nixal_reprap_XmotorCompatible (Autodesk Fusion 360 design; units mm, degrees)
Autodesk Fusion 360 part; units mm, degrees
sketch "Sketch1" plane through (0, 0, 0) normal (0, 1, 0) x (1, 0, 0)
  circle A0 centre (0, 0) radius 4
  circle A1 centre (21, -2) radius 4
  circle A2 centre (21, -2) radius 13
  circle A3 centre (21, -2) radius 8 construction
  circle A4 centre (13, -1.9989) radius 1.8
  circle A5 centre (29, -2.0036) radius 1.8
  line L0 (21, -2) -> (21, 11) construction
  line L1 (21, -2) -> (34, -2) construction
  line L2 (41, 31) -> (-24, 31)
  line L3 (41, 31) -> (41, -15)
  circle A6 centre (0, 0) radius 6
  circle A7 centre (0, 0) radius 10.5
  line L4 (40.8805, 9) -> (-49.1195, 9)
  line L5 (-49.1195, 9) -> (-49.1195, 26)
  line L6 (-49.1195, 26) -> (40.8805, 26)
  line L7 (40.8805, 26) -> (40.8805, 9)
  line L8 (-10.5, 0.0002) -> (-10.4998, 9)
  line L9 (34, -2) -> (34, 9)
  line L10 (0, 0) -> (7.1243, -7.7132)
  line L11 (0, 0) -> (6, -9)
  circle A8 centre (21, -2) radius 5.5
  line L12 (10.5, 0.0203) -> (10.4826, 9)
  line L13 (7.1243, -7.7132) -> (14.0549, -12.9894)
  circle A9 centre (21, 6) radius 1.8
  circle A10 centre (20.9776, -10) radius 1.8
  dimension "d1" = 8
  dimension "d2" = 8
  dimension "d23" = 26
  dimension "d104" = 16
  dimension "d107" = 3.6
  dimension "d108" = 3.6
  dimension "d134" = 33
  dimension "d136" = 31
  dimension "d137" = 20
  dimension "d138" = 41
  dimension "d139" = 12
  dimension "d140" = 21
  dimension "d141" = 17
  dimension "d142" = 90
  dimension "d143" = 5
  dimension "d146" = 11
  dimension "d203" = 3.6
  dimension "d204" = 3.6
  constraint coincident A0.centre A6.centre
  constraint concentric A1 A2
  constraint coincident A3 A0.centre
  constraint coincident A3
  constraint coincident A2 A0.centre
  constraint vertical L0
  constraint horizontal L1
  constraint horizontal L2
  constraint vertical L3
  constraint concentric A0 A6
  constraint concentric A6 A7
  constraint horizontal L4
  constraint vertical L5
  constraint horizontal L6
  constraint vertical L7
  constraint coincident A7 A0.centre
  constraint coincident L4
  constraint tangent A7 L8
  constraint tangent A2 L9
  constraint concentric A3 A8
  constraint tangent A7 L12
  constraint coincident L0 A0.centre
  measures "d1" diameter of A0
  measures "d2" diameter of A1
  measures "d23" diameter of A2
  measures "d104" diameter of A3
  measures "d107" diameter of A4
  measures "d108" diameter of A5
  measures "d134" distance of A0.centre L2
  measures "d136" distance of A0.centre L2
  measures "d137" distance of A0.centre L3
  measures "d138" distance of A0.centre L3
  measures "d139" diameter of A6
  measures "d140" diameter of A7
  measures "d143" distance of L2 L6
  measures "d146" diameter of A8
  measures "d203" diameter of A9
  measures "d204" diameter of A10
extrude "Extrude24" add sketch "Sketch1" along normal blind 62 contours A2 A6 A7 L4 L10 L11 | A7 L4 L8 | A2 A7 | A2 A7 L4 L5 L6 L7 | A7 L4 | A2 A7 L4 L12 | A2 A7 L12 | A2 L4
extrude "Extrude26" add sketch "Sketch1" along normal blind 62 and the other way blind -54 contours A2 A7 L13 | A2 A7 L4 L12 L13 | A2 L4 L12 | A2 L4 L9
sketch "Sketch7" plane through (40.8805, 0, 0) normal (1, 0, 0) x (0, 0, -1)
  line L0 (9, 0) -> (26, 0)
  line L1 (26, 0) -> (26, 62)
  line L2 (26, 62) -> (9, 62)
  line L3 (9, 62) -> (9, 0)
  line L4 (9, 62) -> (26, 0) construction
  line L5 (9, 0) -> (26, 62) construction
  line L6 (17.5, 31) -> (17.5, 53.5) construction
  line L7 (17.5, 31) -> (17.5, 8.5) construction
  circle A0 centre (17.5, 53.5) radius 6
  circle A1 centre (17.5, 8.5) radius 6
  line L8 (23, 46) -> (12, 46)
  line L9 (12, 46) -> (12, 16)
  line L10 (12, 16) -> (23, 16)
  line L11 (23, 16) -> (23, 46)
  line L12 (23, 46) -> (12, 16) construction
  line L13 (12, 46) -> (23, 16) construction
  line L14 (22.7211, 43.5) -> (12.2789, 43.5)
  line L15 (12.2789, 43.5) -> (12.2789, 18.5)
  line L16 (12.2789, 18.5) -> (22.7211, 18.5)
  line L17 (22.7211, 18.5) -> (22.7211, 43.5)
  line L18 (22.7211, 43.5) -> (12.2789, 18.5) construction
  line L19 (12.2789, 43.5) -> (22.7211, 18.5) construction
  dimension "d173" = 22.5
  dimension "d174" = 22.5
  dimension "d175" = 12
  dimension "d176" = 12
  dimension "d179" = 30
  dimension "d180" = 11
  dimension "d195" = 25
  constraint midpoint L4
  constraint perpendicular L8 L9
  constraint parallel L8 L10
  constraint parallel L9 L11
  constraint horizontal L8
  constraint coincident L12
  constraint coincident L13
  constraint perpendicular L14 L15
  constraint parallel L14 L16
  constraint parallel L15 L17
  constraint horizontal L14
  constraint coincident L18
  constraint coincident L19
  measures "d174" distance of origin
  measures "d175" diameter of A0
  measures "d176" diameter of A1
  measures "d179" distance of origin
  measures "d195" distance of origin
extrude "Extrude27" cut sketch "Sketch7" against normal blind 35 contours A0 | A1
extrude "Extrude28" cut sketch "Sketch7" against normal blind 52 contours L8 L9 L10 L11 | L14 L15 L16 L17
sketch "Sketch8" plane through (0, 0, -9) normal (0, 0, 1) x (1, 0, 0)
  line L0 (-49.1195, 0) -> (-10.4998, 0)
  line L1 (-10.4998, 0) -> (-10.4998, 62)
  line L2 (-10.4998, 62) -> (-49.1195, 62)
  line L3 (-49.1195, 62) -> (-49.1195, 0)
  line L4 (-49.1195, 62) -> (-10.4998, 0) construction
  line L5 (-10.4998, 62) -> (-49.1195, 0) construction
  circle A0 centre (-29.8096, 31) radius 15
  line L6 (-14.3096, 47) -> (-45.3096, 47) construction
  line L7 (-45.3096, 47) -> (-45.3096, 15) construction
  line L8 (-45.3096, 15) -> (-14.3096, 15) construction
  line L9 (-14.3096, 15) -> (-14.3096, 47) construction
  line L10 (-14.3096, 47) -> (-45.3096, 15) construction
  line L11 (-45.3096, 47) -> (-14.3096, 15) construction
  circle A1 centre (-45.3096, 47) radius 1.65
  circle A2 centre (-14.3096, 47) radius 1.65
  circle A3 centre (-45.3096, 15) radius 1.65
  circle A4 centre (-14.3096, 15) radius 1.65
  circle A5 centre (-45.3096, 47) radius 3
  circle A6 centre (-14.3096, 47) radius 3
  circle A7 centre (-14.3096, 15) radius 3
  line L12 (-49.1195, 38.5778) -> (-42.7548, 38.5778)
  line L13 (-23, 0) -> (-23, 17.6348)
  line L14 (-49.1195, 62) -> (-10.4998, 62)
  line L15 (-10.4998, 62) -> (-10.4998, 0)
  line L16 (-10.4998, 0) -> (-49.1195, 0)
  line L17 (-49.1195, 0) -> (-49.1195, 62)
  arc A8 (-44.1195, 62) -> (-49.1195, 57) centre (-44.1195, 57) ccw
  dimension "d183" = 30
  dimension "d184" = 31
  dimension "d185" = 32
  dimension "d186" = 3.3
  dimension "d187" = 3.3
  dimension "d188" = 3.3
  dimension "d189" = 3.3
  dimension "d190" = 6
  dimension "d191" = 6
  dimension "d192" = 6
  dimension "d202" = 5
  constraint midpoint L4
  constraint perpendicular L6 L7
  constraint parallel L6 L8
  constraint parallel L7 L9
  constraint horizontal L6
  constraint coincident L10
  constraint coincident L11
  constraint concentric A1 A5
  constraint coincident L3 origin
  constraint perpendicular L7 L12
  constraint coincident A0 origin
  constraint perpendicular L8 L13
  constraint horizontal L14
  constraint vertical L15
  constraint horizontal L16
  constraint vertical L17
  constraint coincident L16 origin
  constraint tangent L14 A8
  constraint tangent L17 A8
  constraint coincident L14
  constraint coincident L17
  measures "d183" diameter of A0
  measures "d185" distance of origin
  measures "d186" diameter of A1
  measures "d187" diameter of A2
  measures "d188" diameter of A3
  measures "d189" diameter of A4
  measures "d190" diameter of A5
  measures "d191" diameter of A6
  measures "d192" diameter of A7
  measures "d202" radius of A8
extrude "Extrude29" cut sketch "Sketch8" against normal blind 40 contours L0 L3 A0 L12 L13 L16 L17 | A0 | L2 L3 L14 L17 A8 | A3
extrude "Extrude30" cut sketch "Sketch7" against normal blind 65 contours L14 L15 L16 L17
extrude "Extrude31" cut sketch "Sketch8" against normal blind 40 contours A1 | A2 | A4
extrude "Extrude32" cut sketch "Sketch8" against normal blind 9 contours A5 | A6 | A7
equation "d173 = ( 45 / 2 ) * 1 mm"
equation "d174 = ( 45 / 2 ) * 1 mm"
